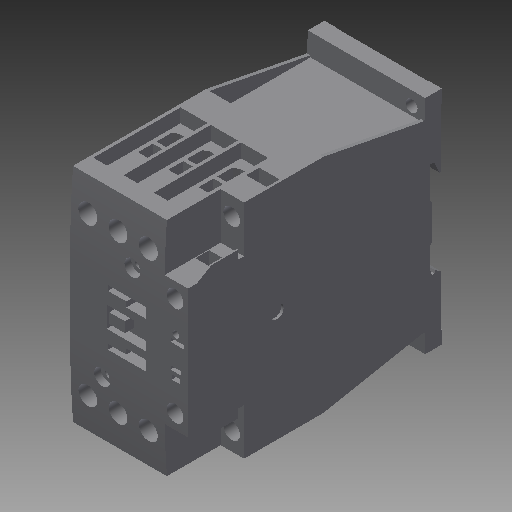
# Autodesk Inventor part: 112442
Saved by Autodesk Inventor 2019.3 (Build 233278000, 278)
## iProperties
Category: PARTsolutions
Company: MOELLER
Created: 2018-10-25
Part Number: 112442
Material: Generic
Catalog Web Link: www.cadenas.de
Description: DC operated-
Vendor: MOELLER
Document SubType Name: Modeling
Designer: psadmin
Manufacturer: MOELLER
Mass: 306.651 g
Surface Area: 470.482 cm^2
Volume: 306.651 cm^3
Density: 1 g/cm^3
Appearance: PSOLRGB-175-175-175
PSOL_IDENT_0: {$CADENAS_DATA\23d-libs\moeller\2\695\733\735\737\740.prj},171 {VTYP=3D},{NB=112442},{LINA=112442},{
PSOL_IDENT_1: NN=DC operated},{DATE=04.10.2018 12:16:44},{GEOMDATE=04.10.2018 08:29:25},{VERSION=v181004082925},{L
PSOL_IDENT_2: INEID=110},{WBVAR=},{WBNUMERIC=}  {NB=112442},{LINA=112442},{KT=DUMMY},{PFOTO=2110pic-213.jpg},{PLID=
PSOL_IDENT_3: 112442},{DATA_SHEET=Data sheet},{MANUTYPEDESC=DILM38-10(RDC24)},{DESCSHORT=Contactor, 3p+1N/O, 18.5k
PSOL_IDENT_4: W/400V/AC3},{DESCLONG=Contactor, Application: Contactors for Motors, Contactors up to 170 A, 3 pole,
PSOL_IDENT_5: Utilization category: AC-1: Non-inductive or slightly inductive loads, resistance furnaces, NAC-3:
PSOL_IDENT_6: Normal AC induction motors: starting, switch off during running, AC-4: Normal AC induction motors: s
PSOL_IDENT_7: tarting, plugging, reversing, inching, Connection technique: Screw terminals, Notes: Not suitable fo
PSOL_IDENT_8: r motors with efficiency class IE3., Number of poles: 3 pole, Rated operational current AC-3 380 V 4
PSOL_IDENT_9: 00 V: Ie= 38 A, Rated operational current AC-1 Conventional free air thermal current, 3 pole, 50 - 6
PSOL_IDENT_10: 0 Hz Open at 40 °C: Ith =Ie= 45 A, enclosed: Ith= 36 A, Rated operational current AC-1 Conventional
PSOL_IDENT_11: free air thermal current, 1 pole open: Ith= 100 A, enclosed: Ith= 90 A, Max. rating for three-phase
PSOL_IDENT_12: motors, 50 - 60 Hz AC-3 220 V 230 V: P= 11 kW, 380 V 400 V: P= 18.5 kW, 660 V 690 V: P= 21 kW, Max.
PSOL_IDENT_13: rating for three-phase motors, 50 - 60 Hz AC-4 220 V 230 V: P= 4 kW, 380 V 400 V: P= 7 kW, 660 V 690
PSOL_IDENT_14: V: P= 10 kW, Can be combined with auxiliary contact: DILM32-XHI.., DILA-XHI(V).., DILM32-XHI11-S, C
PSOL_IDENT_15: ontacts N/O = Normally open: 1 N/O, Instructions: Contacts to EN 50 012., integrated suppressor circ
PSOL_IDENT_16: uit in actuating electronics, Voltage AC/DC: DC operation},{EAN=4015081119981},{ECLASS_8_1=27-37-10-
PSOL_IDENT_17: 03},{PACKAGED_WEIGHT=0.534},{DATA_SHEET_=http://datasheet.moeller.net/datasheet.php?model=112442&loc
PSOL_IDENT_18: ale=en_GB},{DATA_SHEET_ENG=http://datasheet.moeller.net/datasheet.php?model=112442&locale=en_GB},{DA
PSOL_IDENT_19: TA_SHEET_DEU=http://datasheet.moeller.net/datasheet.php?model=112442&locale=de_DE}
NN: DC operated
NB: 112442
NBSYN: $PLID.
LINA: 112442
PFOTO: 2110pic-213.jpg
PLID: 112442
DATA_SHEET: Data sheet
MANUTYPEDESC: DILM38-10(RDC24)
DESCSHORT: Contactor, 3p+1N/O, 18.5kW/400V/AC3
DESCLONG: Contactor, Application: Contactors for Motors, Contactors up to 170 A, 3 pole, Utilization category: AC-1: Non-inductive or slightly inductive loads, resistance furnaces, NAC-3: Normal AC induction motors: starting, switch off during running, AC-4: Normal AC induction motors: starting, plugging, reversing, inching, Connection technique: Screw terminals, Notes: Not suitable for motors with efficiency class IE3., Number of poles: 3 pole, Rated operational current AC-3 380 V 400 V: Ie= 38 A, Rated operational current AC-1 Conventional free air thermal current, 3 pole, 50 - 60 Hz Open at 40 °C: Ith =Ie= 45 A, enclosed: Ith= 36 A, Rated operational current AC-1 Conventional free air thermal current, 1 pole open: Ith= 100 A, enclosed: Ith= 90 A, Max. rating for three-phase motors, 50 - 60 Hz AC-3 220 V 230 V: P= 11 kW, 380 V 400 V: P= 18.5 kW, 660 V 690 V: P= 21 kW, Max. rating for three-phase motors, 50 - 60 Hz AC-4 220 V 230 V: P= 4 kW, 380 V 400 V: P= 7 kW, 660 V 690 V: P= 10 kW, Can be combined with auxiliary contact: DILM32-XHI.., DILA-XHI(V).., DILM32-XHI11-S, Contacts N/O = Normally open: 1 N/O, Instructions: Contacts to EN 50 012., integrated suppressor circuit in actuating electronics, Voltage AC/DC: DC operation
EAN: 4015081119981
ECLASS_8_1: 27-37-10-03
PACKAGED_WEIGHT: 0.534
SUPPLIER: MOELLER
ARTICLENO: 112442
BOMINFO: 112442
CREATOR: CADENAS GmbH
Title: 112442
Author: Cadenas PARTsolutions
Autodesk Inventor part; units mm, degrees
sketch "Sketch_1" plane through (0, 0, 0) normal (1, 0, 0) x (0, 1, 0)
  line L0 (12.5, 93.8) -> (-12.5, 93.8)
  arc A0 (-12.5, 93.8) -> (-42.5, 92.701) centre (-12.5, -316.2) ccw
  line L1 (-42.5, 92.701) -> (-42.5, 41.7)
  line L2 (-42.5, 41.7) -> (-34.9953, 2.9761)
  line L3 (-34.9953, 2.9761) -> (-42.5, 2.714)
  line L4 (-42.5, 2.714) -> (-42.5, -3.7)
  line L5 (-42.5, -3.7) -> (-18.343, -3.7)
  line L6 (-18.343, -3.7) -> (-16.5, -1.0679)
  line L7 (-16.5, -1.0679) -> (-17.5, -0.8)
  line L8 (-17.5, -0.8) -> (-17.5, 0.1064)
  line L9 (-17.5, 0.1064) -> (-15.0449, 1)
  line L10 (-15.0449, 1) -> (-7.5, 1)
  line L11 (-7.5, 1) -> (-6.5, 0)
  line L12 (-6.5, 0) -> (6.5, 0)
  line L13 (6.5, 0) -> (7.5, 1)
  line L14 (7.5, 1) -> (19.5, 1)
  line L15 (19.5, 1) -> (19.5, -0.7016)
  line L16 (19.5, -0.7016) -> (15, -2.8)
  line L17 (15, -2.8) -> (15, -3.7)
  line L18 (15, -3.7) -> (42.5, -3.7)
  line L19 (42.5, -3.7) -> (42.5, 2.714)
  line L20 (42.5, 2.714) -> (34.9953, 2.9761)
  line L21 (34.9953, 2.9761) -> (42.5, 41.7)
  line L22 (42.5, 41.7) -> (42.5, 92.701)
  arc A1 (42.5, 92.701) -> (12.5, 93.8) centre (12.5, -316.2) ccw
  constraints: 46 end point, 4 point on circle, 2 centre point
extrude "Extrusion1" add sketch "Sketch_1" along normal blind 45
sketch "Sketch_84" plane through (0, 0, -3.7) normal (0, 0, 1) x (1, 0, 0)
  line L0 (0, 37.5) -> (0, -37.5)
  line L1 (0, -37.5) -> (1.2, -37.5)
  line L2 (1.2, -37.5) -> (1.2, -41.3)
  line L3 (1.2, -41.3) -> (5, -41.3)
  line L4 (5, -41.3) -> (5, -42.5)
  line L5 (5, -42.5) -> (40, -42.5)
  line L6 (40, -42.5) -> (40, -41.3)
  line L7 (40, -41.3) -> (43.8, -41.3)
  line L8 (43.8, -41.3) -> (43.8, -37.5)
  line L9 (43.8, -37.5) -> (45, -37.5)
  line L10 (45, -37.5) -> (45, 37.5)
  line L11 (45, 37.5) -> (43.8, 37.5)
  line L12 (43.8, 37.5) -> (43.8, 41.3)
  line L13 (43.8, 41.3) -> (40, 41.3)
  line L14 (40, 41.3) -> (40, 42.5)
  line L15 (40, 42.5) -> (5, 42.5)
  line L16 (5, 42.5) -> (5, 41.3)
  line L17 (5, 41.3) -> (1.2, 41.3)
  line L18 (1.2, 41.3) -> (1.2, 37.5)
  line L19 (1.2, 37.5) -> (0, 37.5)
  constraints: 40 end point
extrude "Extrusion2" cut sketch "Sketch_84" along normal blind 0.2
sketch "Sketch_2" plane through (36, 0, 0) normal (1, 0, 0) x (0, 0, -1)
  line L0 (-102.1, -42.5) -> (-72.1, -42.5)
  line L1 (-72.1, -42.5) -> (-72.1, -24.7)
  line L2 (-72.1, -24.7) -> (-101.1, -24.7)
  line L3 (-101.1, -24.7) -> (-101.1, 24.7)
  line L4 (-101.1, 24.7) -> (-72.1, 24.7)
  line L5 (-72.1, 24.7) -> (-72.1, 42.5)
  line L6 (-72.1, 42.5) -> (-102.1, 42.5)
  line L7 (-102.1, 42.5) -> (-102.1, -42.5)
  constraints: 16 end point
extrude "Extrusion3" cut sketch "Sketch_2" along normal blind 10
sketch "Sketch_87" plane through (45, 0, 0) normal (1, 0, 0) x (0, 0, -1)
  line L0 (-90.3, 24.7) -> (-90.3, -24.7)
  line L1 (-90.3, -24.7) -> (-84.5842, -28)
  line L2 (-84.5842, -28) -> (-74.3, -28)
  line L3 (-74.3, -28) -> (-74.3, 28)
  line L4 (-74.3, 28) -> (-84.5842, 28)
  line L5 (-84.5842, 28) -> (-90.3, 24.7)
  constraints: 12 end point
extrude "Extrusion4" add sketch "Sketch_87" against normal blind 0.5
sketch "Sketch_4" plane through (22.5, 0, 0) normal (1, 0, 0) x (0, 0, -1)
  line L0 (-41.7, 34.3) -> (-3.0004, 34.3)
  line L1 (-3.0004, 34.3) -> (-2.714, 42.5)
  line L2 (-2.714, 42.5) -> (-41.7, 42.5)
  line L3 (-41.7, 42.5) -> (-41.7, 34.3)
  constraints: 8 end point
extrude "Extrusion5" cut sketch "Sketch_4" along normal mid plane 42.4
sketch "Sketch_3" plane through (22.5, 0, 0) normal (1, 0, 0) x (0, 0, -1)
  line L0 (-41.7, -34.3) -> (-41.7, -42.5)
  line L1 (-41.7, -42.5) -> (-2.714, -42.5)
  line L2 (-2.714, -42.5) -> (-3.0004, -34.3)
  line L3 (-3.0004, -34.3) -> (-41.7, -34.3)
  constraints: 8 end point
extrude "Extrusion6" cut sketch "Sketch_3" along normal mid plane 42.4
sketch "Sketch_5" plane through (0, 0, 93.8) normal (0, 0, 1) x (1, 0, 0)
  line L0 (14, 4) -> (14, -4)
  line L1 (14, -4) -> (29, -4)
  line L2 (29, -4) -> (29, 4)
  line L3 (29, 4) -> (14, 4)
  line L4 (15, -1.95) -> (21, -1.95)
  line L5 (21, -1.95) -> (21, 1.95)
  line L6 (21, 1.95) -> (15, 1.95)
  line L7 (15, 1.95) -> (15, -1.95)
  constraints: 16 end point
extrude "Extrusion7" cut sketch "Sketch_5" against normal blind 3.5
sketch "Sketch_6" plane through (0, 0, 93.8) normal (0, 0, 1) x (1, 0, 0)
  line L0 (14.5, 8.8) -> (21.5, 8.8)
  line L1 (21.5, 8.8) -> (21.5, 6.8)
  line L2 (21.5, 6.8) -> (29, 6.8)
  line L3 (29, 6.8) -> (29, 10.725)
  line L4 (29, 10.725) -> (14.5, 10.725)
  line L5 (14.5, 10.725) -> (14.5, 8.8)
  constraints: 12 end point
extrude "Extrusion8" cut sketch "Sketch_6" against normal blind 4
sketch "Sketch_7" plane through (0, 0, 93.8) normal (0, 0, 1) x (1, 0, 0)
  line L0 (14.5, -8.8) -> (14.5, -10.725)
  line L1 (14.5, -10.725) -> (29, -10.725)
  line L2 (29, -10.725) -> (29, -6.8)
  line L3 (29, -6.8) -> (21.5, -6.8)
  line L4 (21.5, -6.8) -> (21.5, -8.8)
  line L5 (21.5, -8.8) -> (14.5, -8.8)
  constraints: 12 end point
extrude "Extrusion9" cut sketch "Sketch_7" against normal blind 4
sketch "Sketch_8" plane through (0, 0, 84.31) normal (0, 0, 1) x (1, 0, 0)
  circle A0 centre (6.4, 30.2) radius 3.6
  constraints: 1 centre point
extrude "Extrusion10" cut sketch "Sketch_8" along normal blind 10
sketch "Sketch_9" plane through (0, 0, 84.31) normal (0, 0, 1) x (1, 0, 0)
  circle A0 centre (18, 30.2) radius 3.6
  constraints: 1 centre point
extrude "Extrusion11" cut sketch "Sketch_9" along normal blind 10
sketch "Sketch_10" plane through (0, 0, 84.31) normal (0, 0, 1) x (1, 0, 0)
  circle A0 centre (29.6, 30.2) radius 3.6
  constraints: 1 centre point
extrude "Extrusion12" cut sketch "Sketch_10" along normal blind 10
sketch "Sketch_11" plane through (0, 0, 84.31) normal (0, 0, 1) x (1, 0, 0)
  circle A0 centre (29.6, -30.2) radius 3.6
  constraints: 1 centre point
extrude "Extrusion13" cut sketch "Sketch_11" along normal blind 10
sketch "Sketch_12" plane through (0, 0, 84.31) normal (0, 0, 1) x (1, 0, 0)
  circle A0 centre (18, -30.2) radius 3.6
  constraints: 1 centre point
extrude "Extrusion14" cut sketch "Sketch_12" along normal blind 10
sketch "Sketch_13" plane through (0, 0, 84.31) normal (0, 0, 1) x (1, 0, 0)
  circle A0 centre (6.4, -30.2) radius 3.6
  constraints: 1 centre point
extrude "Extrusion15" cut sketch "Sketch_13" along normal blind 10
sketch "Sketch_14" plane through (0, 0, 84.31) normal (0, 0, 1) x (1, 0, 0)
  circle A0 centre (6.4, 30.2) radius 4
  line L0 (4.025, 29.65) -> (5.85, 29.65)
  line L1 (5.85, 29.65) -> (5.85, 26.6)
  line L2 (5.85, 26.6) -> (6.95, 26.6)
  line L3 (6.95, 26.6) -> (6.95, 29.65)
  line L4 (6.95, 29.65) -> (8.775, 29.65)
  line L5 (8.775, 29.65) -> (8.775, 30.75)
  line L6 (8.775, 30.75) -> (6.95, 30.75)
  line L7 (6.95, 30.75) -> (6.95, 33.8)
  line L8 (6.95, 33.8) -> (5.85, 33.8)
  line L9 (5.85, 33.8) -> (5.85, 30.75)
  line L10 (5.85, 30.75) -> (4.025, 30.75)
  line L11 (4.025, 30.75) -> (4.025, 29.65)
  constraints: 24 end point, 1 centre point
extrude "Extrusion16" add sketch "Sketch_14" along normal blind 1.2
sketch "Sketch_15" plane through (0, 0, 84.31) normal (0, 0, 1) x (1, 0, 0)
  circle A0 centre (18, 30.2) radius 4
  line L0 (15.625, 29.65) -> (17.45, 29.65)
  line L1 (17.45, 29.65) -> (17.45, 26.6)
  line L2 (17.45, 26.6) -> (18.55, 26.6)
  line L3 (18.55, 26.6) -> (18.55, 29.65)
  line L4 (18.55, 29.65) -> (20.375, 29.65)
  line L5 (20.375, 29.65) -> (20.375, 30.75)
  line L6 (20.375, 30.75) -> (18.55, 30.75)
  line L7 (18.55, 30.75) -> (18.55, 33.8)
  line L8 (18.55, 33.8) -> (17.45, 33.8)
  line L9 (17.45, 33.8) -> (17.45, 30.75)
  line L10 (17.45, 30.75) -> (15.625, 30.75)
  line L11 (15.625, 30.75) -> (15.625, 29.65)
  constraints: 24 end point, 1 centre point
extrude "Extrusion17" add sketch "Sketch_15" along normal blind 1.2
sketch "Sketch_16" plane through (0, 0, 84.31) normal (0, 0, 1) x (1, 0, 0)
  circle A0 centre (29.6, 30.2) radius 4
  line L0 (27.225, 29.65) -> (29.05, 29.65)
  line L1 (29.05, 29.65) -> (29.05, 26.6)
  line L2 (29.05, 26.6) -> (30.15, 26.6)
  line L3 (30.15, 26.6) -> (30.15, 29.65)
  line L4 (30.15, 29.65) -> (31.975, 29.65)
  line L5 (31.975, 29.65) -> (31.975, 30.75)
  line L6 (31.975, 30.75) -> (30.15, 30.75)
  line L7 (30.15, 30.75) -> (30.15, 33.8)
  line L8 (30.15, 33.8) -> (29.05, 33.8)
  line L9 (29.05, 33.8) -> (29.05, 30.75)
  line L10 (29.05, 30.75) -> (27.225, 30.75)
  line L11 (27.225, 30.75) -> (27.225, 29.65)
  constraints: 24 end point, 1 centre point
extrude "Extrusion18" add sketch "Sketch_16" along normal blind 1.2
sketch "Sketch_17" plane through (0, 0, 84.31) normal (0, 0, 1) x (1, 0, 0)
  circle A0 centre (29.6, -30.2) radius 4
  line L0 (27.225, -30.75) -> (29.05, -30.75)
  line L1 (29.05, -30.75) -> (29.05, -33.8)
  line L2 (29.05, -33.8) -> (30.15, -33.8)
  line L3 (30.15, -33.8) -> (30.15, -30.75)
  line L4 (30.15, -30.75) -> (31.975, -30.75)
  line L5 (31.975, -30.75) -> (31.975, -29.65)
  line L6 (31.975, -29.65) -> (30.15, -29.65)
  line L7 (30.15, -29.65) -> (30.15, -26.6)
  line L8 (30.15, -26.6) -> (29.05, -26.6)
  line L9 (29.05, -26.6) -> (29.05, -29.65)
  line L10 (29.05, -29.65) -> (27.225, -29.65)
  line L11 (27.225, -29.65) -> (27.225, -30.75)
  constraints: 24 end point, 1 centre point
extrude "Extrusion19" add sketch "Sketch_17" along normal blind 1.2
sketch "Sketch_18" plane through (0, 0, 84.31) normal (0, 0, 1) x (1, 0, 0)
  circle A0 centre (18, -30.2) radius 4
  line L0 (15.625, -30.75) -> (17.45, -30.75)
  line L1 (17.45, -30.75) -> (17.45, -33.8)
  line L2 (17.45, -33.8) -> (18.55, -33.8)
  line L3 (18.55, -33.8) -> (18.55, -30.75)
  line L4 (18.55, -30.75) -> (20.375, -30.75)
  line L5 (20.375, -30.75) -> (20.375, -29.65)
  line L6 (20.375, -29.65) -> (18.55, -29.65)
  line L7 (18.55, -29.65) -> (18.55, -26.6)
  line L8 (18.55, -26.6) -> (17.45, -26.6)
  line L9 (17.45, -26.6) -> (17.45, -29.65)
  line L10 (17.45, -29.65) -> (15.625, -29.65)
  line L11 (15.625, -29.65) -> (15.625, -30.75)
  constraints: 24 end point, 1 centre point
extrude "Extrusion20" add sketch "Sketch_18" along normal blind 1.2
sketch "Sketch_19" plane through (0, 0, 84.31) normal (0, 0, 1) x (1, 0, 0)
  circle A0 centre (6.4, -30.2) radius 4
  line L0 (4.025, -30.75) -> (5.85, -30.75)
  line L1 (5.85, -30.75) -> (5.85, -33.8)
  line L2 (5.85, -33.8) -> (6.95, -33.8)
  line L3 (6.95, -33.8) -> (6.95, -30.75)
  line L4 (6.95, -30.75) -> (8.775, -30.75)
  line L5 (8.775, -30.75) -> (8.775, -29.65)
  line L6 (8.775, -29.65) -> (6.95, -29.65)
  line L7 (6.95, -29.65) -> (6.95, -26.6)
  line L8 (6.95, -26.6) -> (5.85, -26.6)
  line L9 (5.85, -26.6) -> (5.85, -29.65)
  line L10 (5.85, -29.65) -> (4.025, -29.65)
  line L11 (4.025, -29.65) -> (4.025, -30.75)
  constraints: 24 end point, 1 centre point
extrude "Extrusion21" add sketch "Sketch_19" along normal blind 1.2
sketch "Sketch_20" plane through (0, 0, 59.85) normal (0, 0, 1) x (1, 0, 0)
  circle A0 centre (40.2, 35.5) radius 3.2
  constraints: 1 centre point
extrude "Extrusion22" cut sketch "Sketch_20" along normal blind 18
sketch "Sketch_21" plane through (0, 0, 59.85) normal (0, 0, 1) x (1, 0, 0)
  circle A0 centre (40.2, -35.5) radius 3.2
  constraints: 1 centre point
extrude "Extrusion23" cut sketch "Sketch_21" along normal blind 18
sketch "Sketch_22" plane through (0, 0, 62.85) normal (0, 0, 1) x (1, 0, 0)
  arc A0 (37.0899, 36) -> (37.0899, 35) centre (40.2, 35.5) ccw
  line L0 (37.0899, 35) -> (39.7, 35)
  line L1 (39.7, 35) -> (39.7, 33.325)
  line L2 (39.7, 33.325) -> (40.7, 33.325)
  line L3 (40.7, 33.325) -> (40.7, 35)
  line L4 (40.7, 35) -> (43.3101, 35)
  arc A1 (43.3101, 35) -> (43.3101, 36) centre (40.2, 35.5) ccw
  line L5 (43.3101, 36) -> (40.7, 36)
  line L6 (40.7, 36) -> (40.7, 37.675)
  line L7 (40.7, 37.675) -> (39.7, 37.675)
  line L8 (39.7, 37.675) -> (39.7, 36)
  line L9 (39.7, 36) -> (37.0899, 36)
  constraints: 20 end point, 4 point on circle, 2 centre point
sketch "Sketch_24" plane through (0, 0, 79.25) normal (0, 0, 1) x (1, 0, 0)
  circle A0 centre (40.2, 19) radius 3.2
  constraints: 1 centre point
extrude "Extrusion24" cut sketch "Sketch_24" along normal blind 18
sketch "Sketch_25" plane through (0, 0, 79.25) normal (0, 0, 1) x (1, 0, 0)
  circle A0 centre (40.2, -19) radius 3.2
  constraints: 1 centre point
extrude "Extrusion25" cut sketch "Sketch_25" along normal blind 18
sketch "Sketch_26" plane through (0, 0, 82.25) normal (0, 0, 1) x (1, 0, 0)
  arc A0 (37.0899, 19.5) -> (37.0899, 18.5) centre (40.2, 19) ccw
  line L0 (37.0899, 18.5) -> (39.7, 18.5)
  line L1 (39.7, 18.5) -> (39.7, 16.825)
  line L2 (39.7, 16.825) -> (40.7, 16.825)
  line L3 (40.7, 16.825) -> (40.7, 18.5)
  line L4 (40.7, 18.5) -> (43.3101, 18.5)
  arc A1 (43.3101, 18.5) -> (43.3101, 19.5) centre (40.2, 19) ccw
  line L5 (43.3101, 19.5) -> (40.7, 19.5)
  line L6 (40.7, 19.5) -> (40.7, 21.175)
  line L7 (40.7, 21.175) -> (39.7, 21.175)
  line L8 (39.7, 21.175) -> (39.7, 19.5)
  line L9 (39.7, 19.5) -> (37.0899, 19.5)
  constraints: 20 end point, 4 point on circle, 2 centre point
sketch "Sketch_28" plane through (0, 0, 93.8) normal (0, 0, 1) x (1, 0, 0)
  line L0 (38.5, 5.3) -> (38.5, 3.9)
  line L1 (38.5, 3.9) -> (43.6, 3.9)
  line L2 (43.6, 3.9) -> (43.6, 5.3)
  line L3 (43.6, 5.3) -> (38.5, 5.3)
  constraints: 8 end point
extrude "Extrusion26" cut sketch "Sketch_28" against normal blind 2.3
sketch "Sketch_29" plane through (0, 0, 93.8) normal (0, 0, 1) x (1, 0, 0)
  line L0 (38.5, -3.9) -> (38.5, -5.3)
  line L1 (38.5, -5.3) -> (42.5, -5.3)
  line L2 (42.5, -5.3) -> (42.5, -3.9)
  line L3 (42.5, -3.9) -> (38.5, -3.9)
  constraints: 8 end point
extrude "Extrusion27" cut sketch "Sketch_29" against normal blind 12.6
sketch "Sketch_30" plane through (0, 0, 93.8) normal (0, 0, 1) x (1, 0, 0)
  line L0 (39, -6.7) -> (39, -8.4)
  line L1 (39, -8.4) -> (42, -8.4)
  line L2 (42, -8.4) -> (42, -6.7)
  line L3 (42, -6.7) -> (39, -6.7)
  constraints: 8 end point
extrude "Extrusion28" cut sketch "Sketch_30" against normal blind 12.6
sketch "Sketch31" plane through (0, -12.5, 93.8) normal (0, 0, 1) x (1, 0, 0)
  point P0 (40.5, 19.8)
hole "Hole1" at (40.5, 7.3, 93.8) direction (0, 0, -1) diameter 2.58 depth 12.6
sketch "Sketch_32" plane through (0, 0, 93.8) normal (0, 0, 1) x (1, 0, 0)
  circle A0 centre (23.8, 21) radius 3.1
  constraints: 1 centre point
extrude "Extrusion29" cut sketch "Sketch_32" against normal blind 2.7
sketch "Sketch_33" plane through (0, 0, 93.8) normal (0, 0, 1) x (1, 0, 0)
  circle A0 centre (23.8, 21) radius 1.6
  constraints: 1 centre point
extrude "Extrusion30" cut sketch "Sketch_33" against normal blind 7
sketch "Sketch_34" plane through (0, 0, 93.8) normal (0, 0, 1) x (1, 0, 0)
  circle A0 centre (12.2, -21) radius 3.1
  constraints: 1 centre point
extrude "Extrusion31" cut sketch "Sketch_34" against normal blind 2.7
sketch "Sketch_35" plane through (0, 0, 93.8) normal (0, 0, 1) x (1, 0, 0)
  circle A0 centre (12.2, -21) radius 1.6
  constraints: 1 centre point
extrude "Extrusion32" cut sketch "Sketch_35" against normal blind 7
sketch "Sketch_36" plane through (0, 37.2, 0) normal (0, 1, 0) x (1, 0, 0)
  line L0 (1.2, -52.7) -> (1.2, -86.1)
  line L1 (1.2, -86.1) -> (11.6, -86.1)
  line L2 (11.6, -86.1) -> (11.6, -52.7)
  line L3 (11.6, -52.7) -> (1.2, -52.7)
  constraints: 8 end point
extrude "Extrusion33" cut sketch "Sketch_36" along normal blind 7
sketch "Sketch_37" plane through (0, 37.2, 0) normal (0, 1, 0) x (1, 0, 0)
  line L0 (12.8, -52.7) -> (12.8, -86.1)
  line L1 (12.8, -86.1) -> (23.2, -86.1)
  line L2 (23.2, -86.1) -> (23.2, -52.7)
  line L3 (23.2, -52.7) -> (12.8, -52.7)
  constraints: 8 end point
extrude "Extrusion34" cut sketch "Sketch_37" along normal blind 7
sketch "Sketch_38" plane through (0, 37.2, 0) normal (0, 1, 0) x (1, 0, 0)
  line L0 (24.4, -52.7) -> (24.4, -86.1)
  line L1 (24.4, -86.1) -> (34.8, -86.1)
  line L2 (34.8, -86.1) -> (34.8, -52.7)
  line L3 (34.8, -52.7) -> (24.4, -52.7)
  constraints: 8 end point
extrude "Extrusion35" cut sketch "Sketch_38" along normal blind 7
sketch "Sketch_39" plane through (0, -37.2, 0) normal (0, 1, 0) x (1, 0, 0)
  line L0 (24.4, -52.7) -> (24.4, -86.1)
  line L1 (24.4, -86.1) -> (34.8, -86.1)
  line L2 (34.8, -86.1) -> (34.8, -52.7)
  line L3 (34.8, -52.7) -> (24.4, -52.7)
  constraints: 8 end point
extrude "Extrusion36" cut sketch "Sketch_39" against normal blind 7
sketch "Sketch_40" plane through (0, -37.2, 0) normal (0, 1, 0) x (1, 0, 0)
  line L0 (12.8, -52.7) -> (12.8, -86.1)
  line L1 (12.8, -86.1) -> (23.2, -86.1)
  line L2 (23.2, -86.1) -> (23.2, -52.7)
  line L3 (23.2, -52.7) -> (12.8, -52.7)
  constraints: 8 end point
extrude "Extrusion37" cut sketch "Sketch_40" against normal blind 7
sketch "Sketch_41" plane through (0, -37.2, 0) normal (0, 1, 0) x (1, 0, 0)
  line L0 (1.2, -52.7) -> (1.2, -86.1)
  line L1 (1.2, -86.1) -> (11.6, -86.1)
  line L2 (11.6, -86.1) -> (11.6, -52.7)
  line L3 (11.6, -52.7) -> (1.2, -52.7)
  constraints: 8 end point
extrude "Extrusion38" cut sketch "Sketch_41" against normal blind 7
sketch "Sketch_42" plane through (0, 37.2, 0) normal (0, 1, 0) x (1, 0, 0)
  line L0 (2.651, -57.4002) -> (2.651, -63.3)
  line L1 (2.651, -63.3) -> (10.142, -63.3)
  line L2 (10.142, -63.3) -> (10.142, -57.4002)
  line L3 (10.142, -57.4002) -> (8.143, -56.4)
  line L4 (8.143, -56.4) -> (4.65, -56.4)
  line L5 (4.65, -56.4) -> (2.651, -57.4002)
  constraints: 12 end point
extrude "Extrusion39" cut sketch "Sketch_42" against normal blind 12.2
sketch "Sketch_43" plane through (0, 37.2, 0) normal (0, 1, 0) x (1, 0, 0)
  line L0 (14.251, -57.4002) -> (14.251, -63.3)
  line L1 (14.251, -63.3) -> (21.742, -63.3)
  line L2 (21.742, -63.3) -> (21.742, -57.4002)
  line L3 (21.742, -57.4002) -> (19.743, -56.4)
  line L4 (19.743, -56.4) -> (16.25, -56.4)
  line L5 (16.25, -56.4) -> (14.251, -57.4002)
  constraints: 12 end point
extrude "Extrusion40" cut sketch "Sketch_43" against normal blind 12.2
sketch "Sketch_44" plane through (0, 37.2, 0) normal (0, 1, 0) x (1, 0, 0)
  line L0 (25.851, -57.4002) -> (25.851, -63.3)
  line L1 (25.851, -63.3) -> (33.342, -63.3)
  line L2 (33.342, -63.3) -> (33.342, -57.4002)
  line L3 (33.342, -57.4002) -> (31.343, -56.4)
  line L4 (31.343, -56.4) -> (27.85, -56.4)
  line L5 (27.85, -56.4) -> (25.851, -57.4002)
  constraints: 12 end point
extrude "Extrusion41" cut sketch "Sketch_44" against normal blind 12.2
sketch "Sketch_45" plane through (0, -37.2, 0) normal (0, 1, 0) x (1, 0, 0)
  line L0 (25.851, -57.4002) -> (25.851, -63.3)
  line L1 (25.851, -63.3) -> (33.342, -63.3)
  line L2 (33.342, -63.3) -> (33.342, -57.4002)
  line L3 (33.342, -57.4002) -> (31.343, -56.4)
  line L4 (31.343, -56.4) -> (27.85, -56.4)
  line L5 (27.85, -56.4) -> (25.851, -57.4002)
  constraints: 12 end point
extrude "Extrusion42" cut sketch "Sketch_45" along normal blind 12.2
sketch "Sketch_46" plane through (0, -37.2, 0) normal (0, 1, 0) x (1, 0, 0)
  line L0 (14.251, -57.4002) -> (14.251, -63.3)
  line L1 (14.251, -63.3) -> (21.742, -63.3)
  line L2 (21.742, -63.3) -> (21.742, -57.4002)
  line L3 (21.742, -57.4002) -> (19.743, -56.4)
  line L4 (19.743, -56.4) -> (16.25, -56.4)
  line L5 (16.25, -56.4) -> (14.251, -57.4002)
  constraints: 12 end point
extrude "Extrusion43" cut sketch "Sketch_46" along normal blind 12.2
sketch "Sketch_47" plane through (0, -37.2, 0) normal (0, 1, 0) x (1, 0, 0)
  line L0 (2.651, -57.4002) -> (2.651, -63.3)
  line L1 (2.651, -63.3) -> (10.142, -63.3)
  line L2 (10.142, -63.3) -> (10.142, -57.4002)
  line L3 (10.142, -57.4002) -> (8.143, -56.4)
  line L4 (8.143, -56.4) -> (4.65, -56.4)
  line L5 (4.65, -56.4) -> (2.651, -57.4002)
  constraints: 12 end point
extrude "Extrusion44" cut sketch "Sketch_47" along normal blind 12.2
sketch "Sketch_48" plane through (0, 37.2, 0) normal (0, 1, 0) x (1, 0, 0)
  line L0 (2.651, -64.7) -> (2.651, -70.4)
  line L1 (2.651, -70.4) -> (10.142, -70.4)
  line L2 (10.142, -70.4) -> (10.142, -64.7)
  line L3 (10.142, -64.7) -> (2.651, -64.7)
  constraints: 8 end point
extrude "Extrusion45" cut sketch "Sketch_48" against normal blind 12.2
sketch "Sketch_49" plane through (0, 37.2, 0) normal (0, 1, 0) x (1, 0, 0)
  line L0 (14.251, -64.7) -> (14.251, -70.4)
  line L1 (14.251, -70.4) -> (21.742, -70.4)
  line L2 (21.742, -70.4) -> (21.742, -64.7)
  line L3 (21.742, -64.7) -> (14.251, -64.7)
  constraints: 8 end point
extrude "Extrusion46" cut sketch "Sketch_49" against normal blind 12.2
sketch "Sketch_50" plane through (0, 37.2, 0) normal (0, 1, 0) x (1, 0, 0)
  line L0 (25.851, -64.7) -> (25.851, -70.4)
  line L1 (25.851, -70.4) -> (33.342, -70.4)
  line L2 (33.342, -70.4) -> (33.342, -64.7)
  line L3 (33.342, -64.7) -> (25.851, -64.7)
  constraints: 8 end point
extrude "Extrusion47" cut sketch "Sketch_50" against normal blind 12.2
sketch "Sketch_51" plane through (0, -37.2, 0) normal (0, 1, 0) x (1, 0, 0)
  line L0 (25.851, -64.7) -> (25.851, -70.4)
  line L1 (25.851, -70.4) -> (33.342, -70.4)
  line L2 (33.342, -70.4) -> (33.342, -64.7)
  line L3 (33.342, -64.7) -> (25.851, -64.7)
  constraints: 8 end point
extrude "Extrusion48" cut sketch "Sketch_51" along normal blind 12.2
sketch "Sketch_52" plane through (0, -37.2, 0) normal (0, 1, 0) x (1, 0, 0)
  line L0 (14.251, -64.7) -> (14.251, -70.4)
  line L1 (14.251, -70.4) -> (21.742, -70.4)
  line L2 (21.742, -70.4) -> (21.742, -64.7)
  line L3 (21.742, -64.7) -> (14.251, -64.7)
  constraints: 8 end point
extrude "Extrusion49" cut sketch "Sketch_52" along normal blind 12.2
sketch "Sketch_53" plane through (0, -37.2, 0) normal (0, 1, 0) x (1, 0, 0)
  line L0 (2.651, -64.7) -> (2.651, -70.4)
  line L1 (2.651, -70.4) -> (10.142, -70.4)
  line L2 (10.142, -70.4) -> (10.142, -64.7)
  line L3 (10.142, -64.7) -> (2.651, -64.7)
  constraints: 8 end point
extrude "Extrusion50" cut sketch "Sketch_53" along normal blind 12.2
sketch "Sketch_54" plane through (22.5, 0, 0) normal (1, 0, 0) x (0, 0, -1)
  line L0 (-1, -12.5) -> (-1, -17.5)
  line L1 (-1, -17.5) -> (4, -17.5)
  line L2 (4, -17.5) -> (4, -12.5)
  line L3 (4, -12.5) -> (-1, -12.5)
  constraints: 8 end point
extrude "Extrusion51" cut sketch "Sketch_54" along normal mid plane 15
sketch "Sketch_55" plane through (0, 0, 0) normal (1, 0, 0) x (0, 1, 0)
  line L0 (-18.9, 56) -> (-22.4, 56)
  line L1 (-22.4, 56) -> (-22.4, 52)
  line L2 (-22.4, 52) -> (-18.9, 52)
  line L3 (-18.9, 52) -> (-18.9, 52.75)
  line L4 (-18.9, 52.75) -> (-16.4, 52.75)
  line L5 (-16.4, 52.75) -> (-16.4, 55.25)
  line L6 (-16.4, 55.25) -> (-18.9, 55.25)
  line L7 (-18.9, 55.25) -> (-18.9, 56)
  constraints: 16 end point
extrude "Extrusion52" cut sketch "Sketch_55" along normal blind 2
sketch "Sketch_56" plane through (0, 0, 0) normal (1, 0, 0) x (0, 1, 0)
  line L0 (18.9, 56) -> (18.9, 55.25)
  line L1 (18.9, 55.25) -> (16.4, 55.25)
  line L2 (16.4, 55.25) -> (16.4, 52.75)
  line L3 (16.4, 52.75) -> (18.9, 52.75)
  line L4 (18.9, 52.75) -> (18.9, 52)
  line L5 (18.9, 52) -> (22.4, 52)
  line L6 (22.4, 52) -> (22.4, 56)
  line L7 (22.4, 56) -> (18.9, 56)
  constraints: 16 end point
extrude "Extrusion53" cut sketch "Sketch_56" along normal blind 2
sketch "Sketch_57" plane through (0, 0, 0) normal (1, 0, 0) x (0, 1, 0)
  arc A0 (2.3, 52) -> (-2.3, 52) centre (0, 52) ccw
  line L0 (-2.3, 52) -> (-2.3, 44.2)
  arc A1 (-2.3, 44.2) -> (2.3, 44.2) centre (0, 44.2) ccw
  line L1 (2.3, 44.2) -> (2.3, 52)
  constraints: 4 end point, 4 point on circle, 2 centre point
extrude "Extrusion54" cut sketch "Sketch_57" along normal blind 1
sketch "Sketch58" plane through (45, 0, 0) normal (1, 0, 0) x (0, 0, -1)
  point P0 (-59.5, 0)
hole "Hole2" at (45, 0, 59.5) direction (-1, 0, 0) diameter 5.1 depth 0.9
sketch "Sketch_59" plane through (0, 42.5, 0) normal (0, 1, 0) x (1, 0, 0)
  line L0 (36.3, -57.6) -> (36.3, -62.6)
  line L1 (36.3, -62.6) -> (44.1, -62.6)
  line L2 (44.1, -62.6) -> (44.1, -57.6)
  line L3 (44.1, -57.6) -> (36.3, -57.6)
  constraints: 8 end point
extrude "Extrusion55" cut sketch "Sketch_59" against normal blind 11.5
sketch "Sketch_60" plane through (0, -42.5, 0) normal (0, 1, 0) x (1, 0, 0)
  line L0 (36.3, -57.6) -> (36.3, -62.6)
  line L1 (36.3, -62.6) -> (44.1, -62.6)
  line L2 (44.1, -62.6) -> (44.1, -57.6)
  line L3 (44.1, -57.6) -> (36.3, -57.6)
  constraints: 8 end point
extrude "Extrusion56" cut sketch "Sketch_60" along normal blind 11.5
sketch "Sketch_61" plane through (0, 42.5, 0) normal (0, 1, 0) x (1, 0, 0)
  line L0 (36.3, -76.8) -> (36.3, -82.1)
  line L1 (36.3, -82.1) -> (44.1, -82.1)
  line L2 (44.1, -82.1) -> (44.1, -76.8)
  line L3 (44.1, -76.8) -> (36.3, -76.8)
  constraints: 8 end point
extrude "Extrusion57" cut sketch "Sketch_61" against normal blind 28
sketch "Sketch_62" plane through (0, -42.5, 0) normal (0, 1, 0) x (1, 0, 0)
  line L0 (36.3, -76.8) -> (36.3, -82.1)
  line L1 (36.3, -82.1) -> (44.1, -82.1)
  line L2 (44.1, -82.1) -> (44.1, -76.8)
  line L3 (44.1, -76.8) -> (36.3, -76.8)
  constraints: 8 end point
extrude "Extrusion58" cut sketch "Sketch_62" along normal blind 28
sketch "Sketch_63" plane through (40.2, 0, 0) normal (1, 0, 0) x (0, 0, -1)
  line L0 (-57.6, 35.5) -> (-62.85, 35.5)
  line L1 (-62.85, 35.5) -> (-62.85, 38.3952)
  line L2 (-62.85, 38.3952) -> (-60.45, 38.5)
  line L3 (-60.45, 38.5) -> (-60.45, 37.25)
  line L4 (-60.45, 37.25) -> (-57.6, 37.25)
  line L5 (-57.6, 37.25) -> (-57.6, 35.5)
  line L6 (-57.6, 35.5) -> (-62.85, 35.5)
  constraints: 14 end point
revolve "Revolution1" add sketch "Sketch_63" angle 360 about axis through (40.2, 35.5, 57.6) along (0, 0, -1)
sketch "Sketch_64" plane through (40.2, 0, 0) normal (1, 0, 0) x (0, 0, -1)
  line L0 (-57.6, -35.5) -> (-62.85, -35.5)
  line L1 (-62.85, -35.5) -> (-62.85, -32.6048)
  line L2 (-62.85, -32.6048) -> (-60.45, -32.5)
  line L3 (-60.45, -32.5) -> (-60.45, -33.75)
  line L4 (-60.45, -33.75) -> (-57.6, -33.75)
  line L5 (-57.6, -33.75) -> (-57.6, -35.5)
  line L6 (-57.6, -35.5) -> (-62.85, -35.5)
  constraints: 14 end point
revolve "Revolution2" add sketch "Sketch_64" angle 360 about axis through (40.2, -35.5, 57.6) along (0, 0, -1)
sketch "Sketch_65" plane through (40.2, 0, 0) normal (1, 0, 0) x (0, 0, -1)
  line L0 (-76.8, 19) -> (-82.25, 19)
  line L1 (-82.25, 19) -> (-82.25, 21.8952)
  line L2 (-82.25, 21.8952) -> (-79.85, 22)
  line L3 (-79.85, 22) -> (-79.85, 20.75)
  line L4 (-79.85, 20.75) -> (-76.8, 20.75)
  line L5 (-76.8, 20.75) -> (-76.8, 19)
  line L6 (-76.8, 19) -> (-82.25, 19)
  constraints: 14 end point
revolve "Revolution3" add sketch "Sketch_65" angle 360 about axis through (40.2, 19, 76.8) along (0, 0, -1)
sketch "Sketch_66" plane through (40.2, 0, 0) normal (1, 0, 0) x (0, 0, -1)
  line L0 (-76.8, -19) -> (-82.25, -19)
  line L1 (-82.25, -19) -> (-82.25, -16.1048)
  line L2 (-82.25, -16.1048) -> (-79.85, -16)
  line L3 (-79.85, -16) -> (-79.85, -17.25)
  line L4 (-79.85, -17.25) -> (-76.8, -17.25)
  line L5 (-76.8, -17.25) -> (-76.8, -19)
  line L6 (-76.8, -19) -> (-82.25, -19)
  constraints: 14 end point
revolve "Revolution4" add sketch "Sketch_66" angle 360 about axis through (40.2, -19, 76.8) along (0, 0, -1)
extrude "Extrusion59" cut sketch "Sketch_22" against normal blind 1.2
sketch "Sketch_23" plane through (0, 0, 62.85) normal (0, 0, 1) x (1, 0, 0)
  arc A0 (37.0899, -35) -> (37.0899, -36) centre (40.2, -35.5) ccw
  line L0 (37.0899, -36) -> (39.7, -36)
  line L1 (39.7, -36) -> (39.7, -37.675)
  line L2 (39.7, -37.675) -> (40.7, -37.675)
  line L3 (40.7, -37.675) -> (40.7, -36)
  line L4 (40.7, -36) -> (43.3101, -36)
  arc A1 (43.3101, -36) -> (43.3101, -35) centre (40.2, -35.5) ccw
  line L5 (43.3101, -35) -> (40.7, -35)
  line L6 (40.7, -35) -> (40.7, -33.325)
  line L7 (40.7, -33.325) -> (39.7, -33.325)
  line L8 (39.7, -33.325) -> (39.7, -35)
  line L9 (39.7, -35) -> (37.0899, -35)
  constraints: 20 end point, 4 point on circle, 2 centre point
extrude "Extrusion60" cut sketch "Sketch_23" against normal blind 1.2
extrude "Extrusion61" cut sketch "Sketch_26" against normal blind 1.2
sketch "Sketch_27" plane through (0, 0, 82.25) normal (0, 0, 1) x (1, 0, 0)
  arc A0 (37.0899, -18.5) -> (37.0899, -19.5) centre (40.2, -19) ccw
  line L0 (37.0899, -19.5) -> (39.7, -19.5)
  line L1 (39.7, -19.5) -> (39.7, -21.175)
  line L2 (39.7, -21.175) -> (40.7, -21.175)
  line L3 (40.7, -21.175) -> (40.7, -19.5)
  line L4 (40.7, -19.5) -> (43.3101, -19.5)
  arc A1 (43.3101, -19.5) -> (43.3101, -18.5) centre (40.2, -19) ccw
  line L5 (43.3101, -18.5) -> (40.7, -18.5)
  line L6 (40.7, -18.5) -> (40.7, -16.825)
  line L7 (40.7, -16.825) -> (39.7, -16.825)
  line L8 (39.7, -16.825) -> (39.7, -18.5)
  line L9 (39.7, -18.5) -> (37.0899, -18.5)
  constraints: 20 end point, 4 point on circle, 2 centre point
extrude "Extrusion62" cut sketch "Sketch_27" against normal blind 1.2
sketch "Sketch_67" plane through (0, 0, -1) normal (0, 0, 1) x (1, 0, 0)
  circle A0 centre (5, -37.5) radius 2.25
  constraints: 1 centre point
extrude "Extrusion63" cut sketch "Sketch_67" along normal mid plane 10
sketch "Sketch_68" plane through (0, 0, -1) normal (0, 0, 1) x (1, 0, 0)
  circle A0 centre (40, 37.5) radius 2.25
  constraints: 1 centre point
extrude "Extrusion64" cut sketch "Sketch_68" along normal mid plane 10
sketch "Sketch_69" plane through (0, 30.2, 0) normal (0, 1, 0) x (1, 0, 0)
  line L0 (6.4, -70.4) -> (6.4, -65.71)
  line L1 (6.4, -65.71) -> (8.9, -65.71)
  line L2 (8.9, -65.71) -> (8.9, -70.4)
  line L3 (8.9, -70.4) -> (6.4, -70.4)
  line L4 (6.4, -70.4) -> (6.4, -65.71)
  constraints: 10 end point
revolve "Revolution5" add sketch "Sketch_69" angle 360 about axis through (6.4, 30.2, 70.4) along (0, 0, 1)
sketch "Sketch_70" plane through (0, 30.2, 0) normal (0, 1, 0) x (1, 0, 0)
  line L0 (18, -70.4) -> (18, -65.71)
  line L1 (18, -65.71) -> (20.5, -65.71)
  line L2 (20.5, -65.71) -> (20.5, -70.4)
  line L3 (20.5, -70.4) -> (18, -70.4)
  line L4 (18, -70.4) -> (18, -65.71)
  constraints: 10 end point
revolve "Revolution6" add sketch "Sketch_70" angle 360 about axis through (18, 30.2, 70.4) along (0, 0, 1)
sketch "Sketch_71" plane through (0, 30.2, 0) normal (0, 1, 0) x (1, 0, 0)
  line L0 (29.6, -70.4) -> (29.6, -65.71)
  line L1 (29.6, -65.71) -> (32.1, -65.71)
  line L2 (32.1, -65.71) -> (32.1, -70.4)
  line L3 (32.1, -70.4) -> (29.6, -70.4)
  line L4 (29.6, -70.4) -> (29.6, -65.71)
  constraints: 10 end point
revolve "Revolution7" add sketch "Sketch_71" angle 360 about axis through (29.6, 30.2, 70.4) along (0, 0, 1)
sketch "Sketch_72" plane through (0, -30.2, 0) normal (0, 1, 0) x (1, 0, 0)
  line L0 (29.6, -70.4) -> (29.6, -65.71)
  line L1 (29.6, -65.71) -> (32.1, -65.71)
  line L2 (32.1, -65.71) -> (32.1, -70.4)
  line L3 (32.1, -70.4) -> (29.6, -70.4)
  line L4 (29.6, -70.4) -> (29.6, -65.71)
  constraints: 10 end point
revolve "Revolution8" add sketch "Sketch_72" angle 360 about axis through (29.6, -30.2, 70.4) along (0, 0, 1)
sketch "Sketch_73" plane through (0, -30.2, 0) normal (0, 1, 0) x (1, 0, 0)
  line L0 (18, -70.4) -> (18, -65.71)
  line L1 (18, -65.71) -> (20.5, -65.71)
  line L2 (20.5, -65.71) -> (20.5, -70.4)
  line L3 (20.5, -70.4) -> (18, -70.4)
  line L4 (18, -70.4) -> (18, -65.71)
  constraints: 10 end point
revolve "Revolution9" add sketch "Sketch_73" angle 360 about axis through (18, -30.2, 70.4) along (0, 0, 1)
sketch "Sketch_74" plane through (0, -30.2, 0) normal (0, 1, 0) x (1, 0, 0)
  line L0 (6.4, -70.4) -> (6.4, -65.71)
  line L1 (6.4, -65.71) -> (8.9, -65.71)
  line L2 (8.9, -65.71) -> (8.9, -70.4)
  line L3 (8.9, -70.4) -> (6.4, -70.4)
  line L4 (6.4, -70.4) -> (6.4, -65.71)
  constraints: 10 end point
revolve "Revolution10" add sketch "Sketch_74" angle 360 about axis through (6.4, -30.2, 70.4) along (0, 0, 1)
sketch "Sketch_75" plane through (0, 0, 0) normal (0, 0, 1) x (1, 0, 0)
  circle A0 centre (22.5, 0) radius 3.5
  constraints: 1 centre point
extrude "Extrusion65" add sketch "Sketch_75" against normal blind 0.5
sketch "Sketch_76" plane through (0, 0, 2.2) normal (0, 0, 1) x (1, 0, 0)
  line L0 (10, -42.6) -> (13, -42.6)
  line L1 (13, -42.6) -> (13, -34.3)
  line L2 (13, -34.3) -> (10, -34.3)
  line L3 (10, -34.3) -> (10, -42.6)
  constraints: 8 end point
extrude "Extrusion66" cut sketch "Sketch_76" along normal blind 2
sketch "Sketch_77" plane through (0, 0, 2.2) normal (0, 0, 1) x (1, 0, 0)
  line L0 (32, -42.6) -> (35, -42.6)
  line L1 (35, -42.6) -> (35, -34.3)
  line L2 (35, -34.3) -> (32, -34.3)
  line L3 (32, -34.3) -> (32, -42.6)
  constraints: 8 end point
extrude "Extrusion67" cut sketch "Sketch_77" along normal blind 2
sketch "Sketch_78" plane through (0, 0, 0) normal (1, 0, 0) x (0, 1, 0)
  arc A0 (-1, 62.35) -> (-1, 56.65) centre (-1, 59.5) ccw
  line L0 (-1, 56.65) -> (1, 56.65)
  arc A1 (1, 56.65) -> (1, 62.35) centre (1, 59.5) ccw
  line L1 (1, 62.35) -> (-1, 62.35)
  constraints: 4 end point, 4 point on circle, 2 centre point
extrude "Extrusion68" cut sketch "Sketch_78" along normal blind 1.2
ref_plane "DIL_M17_38_XY" through (0, 0, 0) normal (0, 0, 1) x (1, 0, 0)
ref_plane "DIL_M17_38_YZ" through (0, 0, 0) normal (1, 0, 0) x (0, 1, 0)
ref_plane "DIL_M17_38_ZX" through (0, 0, 0) normal (0, 1, 0) x (0, 0, 1)
ref_plane "TO_DUMMY_XY" through (22.5, 0, -0.5) normal (0, 0, 1) x (1, 0, 0)
ref_plane "TO_DUMMY_YZ" through (22.5, 0, -0.5) normal (1, 0, 0) x (0, 1, 0)
ref_plane "TO_DUMMY_ZX" through (22.5, 0, -0.5) normal (0, 1, 0) x (0, 0, 1)
ref_plane "XHI_XY" through (18, 0, 93.8) normal (0, 0, -1) x (1, 0, 0)
ref_plane "XHI_YZ" through (18, 0, 93.8) normal (1, 0, 0) x (0, -1, 0)
ref_plane "XHI_ZX" through (18, 0, 93.8) normal (0, -1, 0) x (0, 0, -1)
ref_plane "XHI11_S_XY" through (0, 20.65, 54) normal (-1, 0, 0) x (0, 0, -1)
ref_plane "XHI11_S_YZ" through (0, 20.65, 54) normal (0, 0, -1) x (0, -1, 0)
ref_plane "XHI11_S_ZX" through (0, 20.65, 54) normal (0, -1, 0) x (-1, 0, 0)
ref_plane "XMV_XY" through (45, 0, 59.5) normal (1, 0, 0) x (0, 0, -1)
ref_plane "XMV_YZ" through (45, 0, 59.5) normal (0, 0, -1) x (0, 1, 0)
ref_plane "XMV_ZX" through (45, 0, 59.5) normal (0, 1, 0) x (1, 0, 0)
ref_plane "XSP_XY" through (45, 0, 93.8) normal (1, 0, 0) x (0, 0, -1)
ref_plane "XSP_YZ" through (45, 0, 93.8) normal (0, 0, -1) x (0, 1, 0)
ref_plane "XSP_ZX" through (45, 0, 93.8) normal (0, 1, 0) x (1, 0, 0)
ref_plane "to_DIL_K12_XY" through (18, 0, 64.8) normal (0, 1, 0) x (1, 0, 0)
ref_plane "to_DIL_K12_YZ" through (18, 0, 64.8) normal (1, 0, 0) x (0, 0, -1)
ref_plane "to_DIL_K12_ZX" through (18, 0, 64.8) normal (0, 0, -1) x (0, 1, 0)
body "Solid1"
